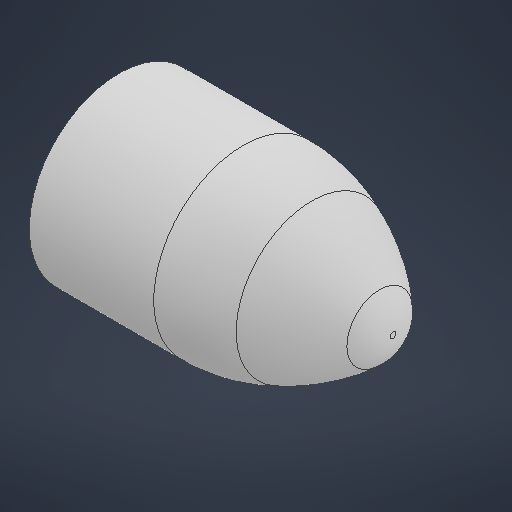
# Autodesk Inventor part: Windmühlen Kopf
Saved by Autodesk Inventor 2026.2 (Build 302298000, 298)
## iProperties
Created: 2026-03-12
Part Number: Windmühlen Kopf
Material: Generic
Document SubType Name: Modeling
Designer: Cobble
Density: 1 g/cm^3
Appearance: Default
Author: Cobble
Autodesk Inventor part; units mm, degrees
ref_plane "YZ Plane" through (0, 0, 0) normal (1, 0, 0) x (0, 1, 0)
ref_plane "XZ Plane" through (0, 0, 0) normal (0, 1, 0) x (-1, 0, 0)
sketch "Sketch1" plane through (0, 0, 0) normal (0, 0, 1) x (1, 0, 0)
  line L0 (0, 0) -> (0, 18)
  line L1 (0, 18) -> (55, 18) construction
  line L2 (55, 18) -> (55, 0) construction
  line L3 (0, 18) -> (55, 18) construction
  line L4 (55, 18) -> (55, -18) construction
  line L5 (55, -18) -> (0, -18) construction
  line L6 (0, -18) -> (0, 18)
  line L7 (0, -12.5) -> (30, -12.5)
  line L8 (30, -12.5) -> (30, 12.5)
  line L9 (30, 12.5) -> (0, 12.5)
  line L10 (55, 0) -> (55, 0.5928)
  line L11 (55, 0) -> (30, 0)
  line L12 (30, 0) -> (30, 18) construction
  arc A0 (52.3154, 6.5716) -> (38.7203, 15.191) centre (19.0942, -30.7961) ccw
  line L13 (0, 18) -> (24.982, 18)
  arc A1 (55, 0.5928) -> (52.3154, 6.5716) centre (47, 0.5928) ccw
  arc A2 (38.7203, 15.191) -> (24.982, 18) centre (24.982, -17) ccw
  line L14 (30, 0) -> (30, 0)
  point P0 (55, 4)
  dimension "d0" = 18
  dimension "d1" = 55
  dimension "d2" = 36
  dimension "d5" = 12.5
  dimension "d6" = 30
  dimension "d7" = 25
  dimension "d14" = 4
  dimension "d16" = 0
  dimension "d17" = 25
  dimension "d18" = 8
  dimension "d19" = 35
  dimension "d20" = 50
  constraints: 30 end point, 8 point on circle, 7 point on line, 4 parallel, 4 perpendicular, 4 tangent, 3 centre point, 3 midpoint, 2 horizontal, 2 vertical
  measures "d0" distance of L0.start L0.end
  measures "d1" distance of L0.end L1.end
  measures "d2" distance of L1.end L4.end
  measures "d5" distance of point (0, 0) L9.end
  measures "d6" distance of L8.end L9.end
  measures "d7" distance of L7.end L8.end
  measures "d14" distance of L2.end point (55, 4)
  measures "d16" distance of L11.start L2.end
  measures "d17" distance of L11.start L11.end
  measures "d18" radius of A1
  measures "d19" radius of A2
  measures "d20" radius of A0
revolve "Revolution1" add sketch "Sketch1" angle 360 about axis through (55, 0, 0) along (-1, 0, 0) contours L0 L13 A2 A0 A1 L10 L11 L8 L9
sketch "Sketch2" plane through (0, 0, 0) normal (-1, 0, 0) x (0, 0, 1)
  circle A0 centre (0, 0) radius 12.5 projected
  circle A1 centre (0, 0) radius 18 projected
  circle A2 centre (0, 0) radius 0.5928 projected
  line L0 (0, 0) -> (0, 12.5)
  circle A3 centre (0, 0) radius 12.5 projected
  circle A4 centre (0, 0) radius 18 projected
  line L1 (0, 12.5) -> (0, 14.5)
  line L2 (0, 14.5) -> (-2.5, 14.5)
  line L3 (0, 14.5) -> (2.5, 14.5)
  line L4 (0, 14.5) -> (0, 12) construction
  line L5 (2.5, 14.5) -> (2.5, 12.2474)
  line L6 (-2.5, 14.5) -> (-2.5, 12.2474)
  point P0 (0, 0)
  point P1 (-2.5, 12.2474)
  point P2 (2.5, 12.2474)
  dimension "d23" = 2
  dimension "d24" = 2.5
  dimension "d25" = 90
  dimension "d26" = 2.5
  dimension "d27" = 90
  constraints: 14 end point, 3 perpendicular, 1 parallel, 1 point on line
  measures "d23" distance of L0.end L1.end
  measures "d24" distance of L1.end L2.end
  measures "d25" angle of L2 L1
  measures "d26" distance of L1.end L3.end
  measures "d27" angle of L4 L3
extrude "Extrusion1" cut sketch "Sketch2" against normal blind 13 contours A0 L1 L3 L5 | L6 L2 L1 A0
ref_plane "Work Plane1" through (0, 18, 0) normal (0, 1, 0) x (-1, 0, 0)
sketch "Sketch3" plane through (0, 18, 0) normal (0, 1, 0) x (-1, 0, 0)
  line L0 (0, -18) -> (0, 18) projected
  line L1 (-24.982, -18) -> (-24.982, 18) projected
  line L2 (-24.982, -18) -> (-24.982, 18) projected
  line L3 (-38.7203, -15.191) -> (-38.7203, 15.191) projected
  line L4 (-38.7203, -15.191) -> (-38.7203, 15.191) projected
  line L5 (-52.3154, -6.5716) -> (-52.3154, 6.5716) projected
  line L6 (-52.3154, -6.5716) -> (-52.3154, 6.5716) projected
  line L7 (-55, -0.5928) -> (-55, 0.5928) projected
  line L8 (0, 0) -> (-11, 0)
  line L9 (-11, 0) -> (-20, 0)
  circle A0 centre (-20, 0) radius 9
  dimension "d30" = 11
  dimension "d31" = 9
  dimension "d42" = 18
  constraints: 4 end point, 2 horizontal, 1 centre point, 1 coincident
  measures "d30" distance of L8.start L8.end
  measures "d31" distance of L8.end L9.end
  measures "d42" diameter of A0
extrude "Extrusion2" cut sketch "Sketch3" against normal blind 3
hole "Hole1" at (20, 18, 0) direction (0, -1, 0) diameter 8.376 depth 18 tip angle 118 thread size "M10x1.5" class "6H" standard "ISO Metric profile"
body "Solid1"
